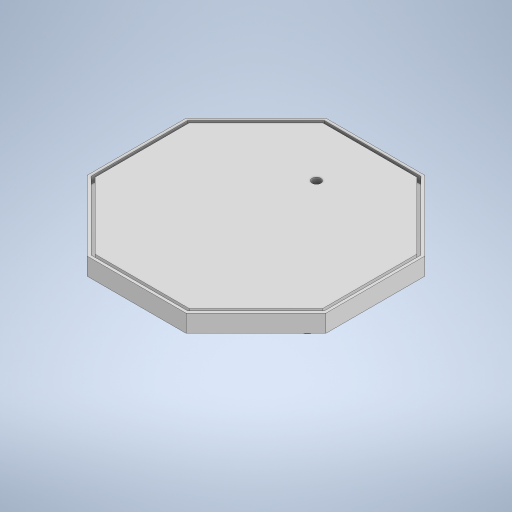
# Autodesk Inventor part: 팔각형 OV-PAM 상단
Saved by Autodesk Inventor 2024 (Build 280153000, 153)
## iProperties
Created: 2023-06-16
Part Number: 팔각형 OV-PAM 상단
Material: 일반
Document SubType Name: Modeling
Designer: jsw
Density: 1 g/cm^3
Appearance: 기본값
Author: jsw
Autodesk Inventor part; units mm, degrees
ref_plane "YZ Plane" through (0, 0, 0) normal (1, 0, 0) x (0, 1, 0)
ref_plane "XZ Plane" through (0, 0, 0) normal (0, 1, 0) x (-1, 0, 0)
ref_plane "XY Plane" through (0, 0, 0) normal (0, 0, 1) x (1, 0, 0)
sketch "스케치3" plane through (0, 0, 0) normal (0, 1, 0) x (-1, 0, 0)
  line L0 (34.1919, -14.1627) -> (14.1627, -34.1919)
  line L1 (14.1627, -34.1919) -> (-14.1627, -34.1919)
  line L2 (-14.1627, -34.1919) -> (-34.1919, -14.1627)
  line L3 (-34.1919, -14.1627) -> (-34.1919, 14.1627)
  line L4 (-34.1919, 14.1627) -> (-14.1627, 34.1919)
  line L5 (-14.1627, 34.1919) -> (14.1627, 34.1919)
  line L6 (14.1627, 34.1919) -> (34.1919, 14.1627)
  line L7 (34.1919, 14.1627) -> (34.1919, -14.1627)
  line L8 (32.5919, -13.5) -> (13.5, -32.5919)
  line L9 (13.5, -32.5919) -> (-13.5, -32.5919)
  line L10 (-13.5, -32.5919) -> (-32.5919, -13.5)
  line L11 (-32.5919, -13.5) -> (-32.5919, 13.5)
  line L12 (-32.5919, 13.5) -> (-13.5, 32.5919)
  line L13 (-13.5, 32.5919) -> (13.5, 32.5919)
  line L14 (13.5, 32.5919) -> (32.5919, 13.5)
  line L15 (32.5919, 13.5) -> (32.5919, -13.5)
  point P0 (0, 0)
  point P1 (0, 0)
  point P2 (0, 0)
  point P3 (0, 0)
  dimension "d43" = 27
  dimension "d44" = 1.6
  constraints: 32 end point, 3 coincident, 2 horizontal, 34 other
  measures "d43" distance of L8.end L9.end
  measures "d44" distance between parallel lines of L7 L15
extrude "돌출2" add sketch "스케치3" along normal blind 5 contours L0 L1 L2 L3 L4 L5 L6 L7 | L8 L9 L10 L11 L12 L13 L14 L15
sketch "스케치4" plane through (0, 5, 0) normal (0, 1, 0) x (1, 0, 0)
  line L0 (13.5, -32.5919) -> (-13.5, -32.5919)
  line L1 (-13.5, -32.5919) -> (-32.5919, -13.5)
  line L2 (-32.5919, -13.5) -> (-32.5919, 13.5)
  line L3 (-32.5919, 13.5) -> (-13.5, 32.5919)
  line L4 (-13.5, 32.5919) -> (13.5, 32.5919)
  line L5 (13.5, 32.5919) -> (32.5919, 13.5)
  line L6 (32.5919, 13.5) -> (32.5919, -13.5)
  line L7 (32.5919, -13.5) -> (13.5, -32.5919)
  line L8 (-13.8314, 33.3919) -> (13.8314, 33.3919)
  line L9 (13.8314, 33.3919) -> (33.3919, 13.8314)
  line L10 (33.3919, 13.8314) -> (33.3919, -13.8314)
  line L11 (33.3919, -13.8314) -> (13.8314, -33.3919)
  line L12 (13.8314, -33.3919) -> (-13.8314, -33.3919)
  line L13 (-13.8314, -33.3919) -> (-33.3919, -13.8314)
  line L14 (-33.3919, -13.8314) -> (-33.3919, 13.8314)
  line L15 (-33.3919, 13.8314) -> (-13.8314, 33.3919)
  point P0 (0, 0)
  point P1 (0, 0)
  point P2 (0, 0)
  dimension "d7" = 27
  dimension "d42" = 0.8
  constraints: 32 end point, 2 coincident, 2 horizontal, 34 other
  measures "d7" distance of L1.end L2.end
  measures "d42" distance between parallel lines of L14 L2
extrude "돌출3" cut sketch "스케치4" against normal blind 2
sketch "스케치5" plane through (0, 0, 0) normal (0, -1, 0) x (1, 0, 0)
  line L0 (10, 2.5) -> (20, 2.5)
  line L1 (20, 2.5) -> (20, -2.5)
  line L2 (20, -2.5) -> (10, -2.5)
  line L3 (10, -2.5) -> (10, 2.5)
  line L4 (10, 2.5) -> (20, -2.5) construction
  line L5 (20, 2.5) -> (10, -2.5) construction
  line L6 (-20, 2.5) -> (-10, 2.5)
  line L7 (-10, 2.5) -> (-10, -2.5)
  line L8 (-10, -2.5) -> (-20, -2.5)
  line L9 (-20, -2.5) -> (-20, 2.5)
  line L10 (-20, 2.5) -> (-10, -2.5) construction
  line L11 (-10, 2.5) -> (-20, -2.5) construction
  point P0 (0, 0)
  point P1 (15, 0)
  point P2 (-15, 0)
  dimension "d11" = 10
  dimension "d12" = 5
  dimension "d13" = 10
  dimension "d16" = 30
  constraints: 24 end point, 2 horizontal, 2 midpoint, 2 parallel, 1 collinear, 1 horizontal alignment, 1 perpendicular, 10 other
  measures "d11" distance of L1.end L2.end
  measures "d12" distance of L0.end L1.end
  measures "d13" distance from line of L3 point (0, 0)
  measures "d16" distance of L0.start L6.start
extrude "돌출4" add sketch "스케치5" along normal blind 10
sketch "스케치6" plane through (-10, 0, -2.5) normal (0, 0, -1) x (-1, 0, 0)
  circle A0 centre (5, -10) radius 5
  circle A1 centre (-25, -10) radius 5
  line L0 (-20, -10) -> (-30, -10) projected
  line L1 (10, -10) -> (0, -10) projected
  point P0 (-10, 0)
  dimension "d23" = 10
  dimension "d24" = 10
  constraints: 2 centre point, 2 coincident, 2 midpoint
  measures "d23" diameter of A0
  measures "d24" diameter of A1
extrude "돌출5" add sketch "스케치6" against normal blind 5
sketch "스케치7" plane through (-10, 0, -2.5) normal (0, 0, -1) x (-1, 0, 0)
  circle A0 centre (5, -10) radius 1.25
  line L0 (10, 0) -> (10, -10) projected
  line L1 (0, 0) -> (10, 0) projected
  line L2 (4.7788, 0) -> (0, 0)
  circle A1 centre (-25, -10) radius 1.25
  point P0 (-10, 0)
  dimension "d27" = 2.5
  dimension "d28" = 5
  dimension "d31" = 30
  constraints: 2 centre point, 2 end point, 1 horizontal, 1 horizontal alignment, 1 point on line, 2 other
  measures "d27" diameter of A0
  measures "d28" distance from line of L0 A0.centre
  measures "d31" distance of A0.centre A1.centre
extrude "돌출6" cut sketch "스케치7" against normal blind 5
sketch "스케치8" plane through (0, 0, 0) normal (0, -1, 0) x (1, 0, 0)
  circle A0 centre (0, -17.3205) radius 1.25
  line L0 (-10, 2.5) -> (-10, -2.5) projected
  point P0 (0, 0)
  point P1 (-10, 0)
  dimension "d38" = 2.5
  dimension "d39" = 17.3205
  constraints: 1 centre point, 1 midpoint, 1 vertical alignment
  measures "d38" diameter of A0
  measures "d39" vertical distance of A0.centre point (-10, 0)
extrude "돌출7" cut sketch "스케치8" against normal blind 5
